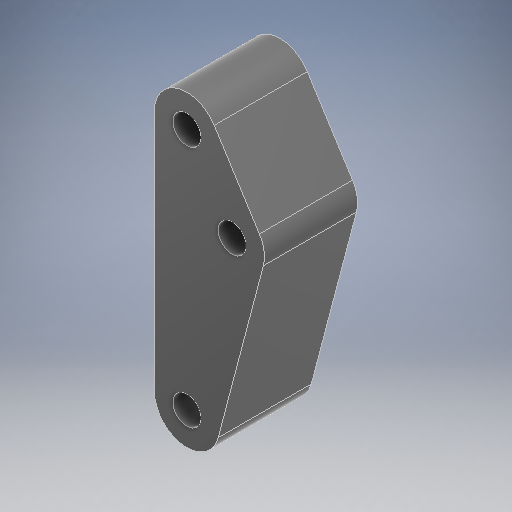
# Autodesk Inventor part: RoundFix
Saved by Autodesk Inventor 2026.1 (Build 301233000, 233)
## iProperties
Created: 2025-10-16
Part Number: RoundFix
Material: Plastic, Opaque Black
Document SubType Name: Modeling
Designer: Teddy
Density: 0.952 g/cm^3
Appearance: Smooth - Black
Author: Teddy
Autodesk Inventor part; units mm, degrees
ref_plane "YZ Plane" through (0, 0, 0) normal (1, 0, 0) x (0, 1, 0)
ref_plane "XZ Plane" through (0, 0, 0) normal (0, 1, 0) x (-1, 0, 0)
ref_plane "XY Plane" through (0, 0, 0) normal (0, 0, 1) x (1, 0, 0)
sketch "Sketch1" plane through (0, 0, 0) normal (0, 0, 1) x (1, 0, 0)
  circle A0 centre (1.1498, 31.75) radius 2.1844 projected
  circle A1 centre (1.1498, -6.35) radius 2.1844 projected
  circle A2 centre (8.2369, 20.5469) radius 2.1844 projected
  arc A3 (-3.9302, -6.35) -> (6.0621, -7.6444) centre (1.1498, -6.35) ccw
  arc A4 (5.4429, 34.4658) -> (-3.9302, 31.75) centre (1.1498, 31.75) ccw
  arc A5 (13.1492, 19.2525) -> (12.53, 23.2627) centre (8.2369, 20.5469) ccw
  line L0 (6.0621, -7.6444) -> (13.1492, 19.2525)
  line L1 (12.53, 23.2627) -> (5.4429, 34.4658)
  line L2 (-3.9302, 31.75) -> (-3.9302, -6.35)
  point P0 (0, 0)
  dimension "d0" = 5.08
  dimension "d1" = 5.08
  dimension "d2" = 5.08
  constraints: 6 end point, 6 point on circle, 5 tangent, 3 centre point, 3 coincident, 1 vertical
  measures "d0" radius of A5
  measures "d1" radius of A4
  measures "d2" radius of A3
extrude "Extrusion1" add sketch "Sketch1" along normal blind 14.605
body "Solid1"
